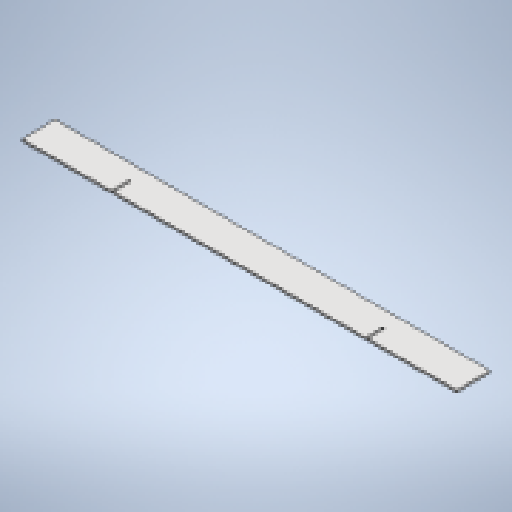
# Autodesk Inventor part: MSC 109 rib cone
Saved by Autodesk Inventor 2025 (Build 290162010, 162A)
## iProperties
Created: 2024-06-26
Part Number: MSC 109 rib cone
Material: Stainless Steel
Document SubType Name: Sheet Metal
Designer: pokla
Density: 8 g/cm^3
Sheet Metal Rule: AISI304 3mm Die 32
Appearance: Default
Stock Number: МОО 109 шпангоут конус
Author: pokla
Autodesk Inventor part; units mm, degrees
ref_plane "YZ Plane" through (0, 0, 0) normal (1, 0, 0) x (0, 1, 0)
ref_plane "XZ Plane" through (0, 0, 0) normal (0, 1, 0) x (-1, 0, 0)
ref_plane "XY Plane" through (0, 0, 0) normal (0, 0, 1) x (1, 0, 0)
sketch "Sketch1" plane through (0, 0, 0) normal (0, 0, 1) x (1, 0, 0)
  line L0 (-400, 50) -> (400, 50)
  line L1 (400, 50) -> (400, 0)
  line L2 (400, 0) -> (-400, 0)
  line L3 (-400, 0) -> (-400, 50)
  circle A0 centre (-400, 0) radius 25
  circle A1 centre (400, 0) radius 25
  point P0 (0, 0)
  point P1 (0, 0)
  point P2 (-400, 25)
  point P3 (-375, 0)
  point P4 (375, 0)
  point P5 (400, 25)
  dimension "d16" = 50
  dimension "d17" = 800
  dimension "d18" = 50
  dimension "d19" = 50
  measures "d16" distance of L0.end L1.end
  measures "d17" distance of L0.start L0.end
  measures "d18" diameter of A0
  measures "d19" diameter of A1
extrude "Plate2" add sketch "Sketch1" against normal blind 3 contours L0 L1 A1 L2 A0 L3 | A0 L2 L3 | L1 L2 A1 picked at (-388.289, 11.711) picked at (398.1457, 16.4577)
sketch "Sketch2" plane through (0, 0, 0) normal (0, 0, 1) x (1, 0, 0)
  line L0 (400, 50) -> (-400, 50) projected
  line L1 (190, 50) -> (190, 0) construction
  line L2 (-400, 0) -> (400, 0) projected
  line L3 (188.5, 26) -> (191.5, 26)
  line L4 (191.5, 26) -> (191.5, 0)
  line L5 (191.5, 0) -> (188.5, 0)
  line L6 (188.5, 0) -> (188.5, 26)
  line L7 (-190, 0) -> (-190, 50) construction
  line L8 (-191.5, 26) -> (-188.5, 26)
  line L9 (-188.5, 26) -> (-188.5, 0)
  line L10 (-188.5, 0) -> (-191.5, 0)
  line L11 (-191.5, 0) -> (-191.5, 26)
  point P0 (0, 0)
  point P1 (0, 0)
  point P2 (188.5, 0)
  point P3 (191.5, 0)
  point P4 (0, 0)
  dimension "d21" = 190
  dimension "d22" = 3
  dimension "d23" = 26
  dimension "d26" = 190
  dimension "d27" = 26
  dimension "d28" = 3
  constraints: 20 end point, 4 midpoint, 4 parallel, 4 point on line, 3 perpendicular, 2 horizontal, 1 vertical
  measures "d21" distance from line of L1 point (0, 0)
  measures "d22" distance of L4.end L5.end
  measures "d23" distance of L3.end L4.end
  measures "d26" distance from line of point (0, 0) L7
  measures "d27" distance of L10.end L8.start
  measures "d28" distance of L9.end L10.end
extrude "Extrusion1" cut sketch "Sketch2" against normal blind 10
sketch "Sketch3" plane through (0, 0, 0) normal (0, 0, 1) x (1, 0, 0)
  line L0 (188.5, 0) -> (188.5, 26) projected
  line L1 (188.5, 26) -> (191.5, 26) projected
  line L2 (191.5, 26) -> (191.5, 0) projected
  line L3 (191.5, 0) -> (400, 0) projected
  line L4 (400, 0) -> (400, 50) projected
  line L5 (400, 50) -> (-400, 50) projected
  line L6 (-400, 50) -> (-400, 0) projected
  line L7 (-400, 0) -> (-191.5, 0) projected
  line L8 (-191.5, 0) -> (-191.5, 26) projected
  line L9 (-191.5, 26) -> (-188.5, 26) projected
  line L10 (-188.5, 26) -> (-188.5, 0) projected
  line L11 (-188.5, 0) -> (188.5, 0) projected
  line L12 (325, 0) -> (325, 50)
  line L13 (400, 50) -> (-400, 50) projected
  line L14 (-325, 0) -> (-325, 50)
  point P0 (0, 0)
  point P1 (325, 50)
  dimension "d29" = 75
  dimension "d30" = 75
  constraints: 4 end point, 4 point on line, 1 parallel, 1 perpendicular
  measures "d29" distance between parallel lines of L4 L12
  measures "d30" distance between parallel lines of L6 L14
extrude "Extrusion2" cut sketch "Sketch3" against normal through all contours L12 L5 L4 L3 | L7 L6 L5 L14
sketch "Sketch4" plane through (0, 0, -3) normal (0, 0, -1) x (-1, 0, 0)
  line L0 (-62.455, 14.7345) -> (-62.455, 33.3208) construction
  line L1 (-62.455, 33.3208) -> (59.5733, 33.3208) construction
  line L2 (59.5733, 33.3208) -> (59.5733, 14.7345) construction
  line L3 (59.5733, 14.7345) -> (-62.455, 14.7345) construction
  point P0 (0, 0)
  constraints: 2 other
mark "Mark1"
equation "\"d22\" = Thickness"
equation "\"d26\" = d21"
equation "\"d27\" = d23"
equation "\"d28\" = Thickness"
equation "\"d30\" = d29"
equation "\"d20\" = Thickness"
equation "\"BendReliefWidth\" = Thickness"
equation "\"BendReliefDepth\" = 0.5 * Thickness"
equation "\"CornerReliefSize\" = 4 * Thickness"
equation "\"MinimumRemnant\" = 2 * Thickness"
equation "\"TransitionRadius\" = BendRadius"
equation "\"JacobiRadiusSize\" = BendRadius"
equation "\"GapSize\" = Thickness"
equation "\"Thickness\" = 3"
equation "\"BendRadius\" = 5"
body "Solid2"
